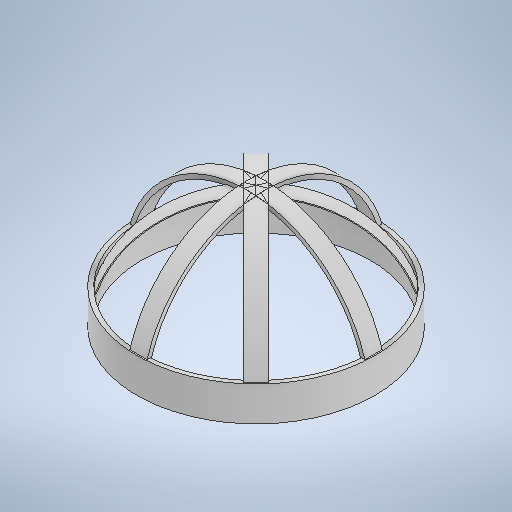
# Autodesk Inventor part: Original Dome
Saved by Autodesk Inventor 2025.1 (Build 291241000, 241)
## iProperties
Created: 2024-11-11
Part Number: Original Dome
Material: Generic
Document SubType Name: Modeling
Designer: monos
Density: 1 g/cm^3
Appearance: Default
Author: monos
Autodesk Inventor part; units mm, degrees
ref_plane "XZ Plane" through (0, 0, 0) normal (0, 1, 0) x (-1, 0, 0)
sketch "Sketch1" plane through (0, 0, 0) normal (0, 1, 0) x (-1, 0, 0)
  circle A0 centre (0, 0) radius 87.5
  circle A1 centre (0, 0) radius 84.325
  dimension "d0" = 175
  dimension "d1" = 168.65
  constraints: 2 centre point, 2 coincident
  measures "d0" diameter of A0
  measures "d1" diameter of A1
extrude "Extrusion1" add sketch "Sketch1" along normal blind 25.4
sketch "Sketch2" plane through (0, 0, 0) normal (1, 0, 0) x (0, 1, 0)
  point P0 (0, 0)
ref_plane "Work Plane1" through (0, 0, 0) normal (0.7071068, 0, -0.7071068) x (0, 1, 0)
sketch "Sketch5" plane through (0, 0, 0) normal (0.7071068, 0, -0.7071068) x (0, 1, 0)
  line L0 (0, -87.5) -> (0, 87.5) projected
  arc A0 (25.4, -86.3414) -> (90, 0) centre (0, 0) ccw
  arc A1 (90, 0) -> (25.4, 86.3414) centre (0, 0) ccw
  arc A2 (25.4, -83.0266) -> (86.825, 0) centre (0, 0) ccw
  arc A3 (86.825, 0) -> (25.4, 83.0266) centre (0, 0) ccw
  line L1 (90, 0) -> (86.825, 0)
  line L2 (25.4187, -86.3359) -> (25.4, -83.0266)
  line L3 (25.4, -87.5) -> (25.4, 87.5) projected
  line L4 (25.4, 83.0266) -> (25.4, 86.3414)
  point P0 (86.825, 0)
  dimension "d13" = 86.825
  dimension "d14" = 86.825
  constraints: 9 point on circle, 6 end point, 4 centre point, 4 coincident, 4 point on line, 1 horizontal
  measures "d13" radius of A2
  measures "d14" radius of A3
extrude "Extrusion4" add sketch "Sketch5" along normal mid plane 12.7 contours L2 A2 L1 A0 | L1 A3 L3 A1
sketch "Sketch3" plane through (0, 0, 0) normal (1, 0, 0) x (0, 1, 0)
  line L0 (0, -87.5) -> (0, 87.5) projected
  arc A0 (90, 0) -> (25.4046, 86.3401) centre (0, 0) ccw
  arc A1 (25.428, -86.3332) -> (90, 0) centre (0, 0) ccw
  arc A2 (25.428, -83.018) -> (86.825, 0) centre (0, 0) ccw
  line L1 (86.825, 0) -> (90, 0)
  line L2 (25.428, -83.018) -> (25.428, -86.3332)
  arc A3 (86.825, 0) -> (25.4046, 83.0252) centre (0, 0) ccw
  line L3 (90, 0) -> (86.825, 0)
  line L4 (25.4046, 86.3401) -> (25.4046, 83.0252)
  dimension "d5" = 86.825
  dimension "d6" = 86.825
  constraints: 8 end point, 8 point on circle, 4 centre point, 4 coincident, 2 horizontal, 1 perpendicular, 1 vertical
  measures "d5" radius of A2
  measures "d6" radius of A3
extrude "Extrusion2" add sketch "Sketch3" along normal mid plane 12.7
sketch "Sketch4" plane through (0, 0, 0) normal (0, 0, 1) x (1, 0, 0)
  line L0 (87.5, 0) -> (-87.5, 0) projected
  arc A0 (0, 90) -> (-86.3414, 25.4) centre (0, 0) ccw
  arc A1 (0, 86.825) -> (-83.0266, 25.4) centre (0, 0) ccw
  arc A2 (83.0266, 25.4) -> (0, 86.825) centre (0, 0) ccw
  line L1 (83.0266, 25.4) -> (86.3414, 25.4)
  line L2 (-86.3414, 25.4) -> (-83.0266, 25.4)
  arc A3 (86.3414, 25.4) -> (0, 90) centre (0, 0) ccw
  line L3 (0, 90) -> (0, 86.825)
  line L4 (0, 90) -> (0, 86.825)
  line L5 (83.0266, 25.4) -> (86.3414, 25.4)
  ellipse E0 centre (4.4901, 0) end of major axis (4.4901, 90) minor radius 63.6396 (-6.35, 88.6847) -> (-56.5586, 25.4187) ccw projected
  line L6 (-83.0266, 25.4) -> (-86.3414, 25.4)
  dimension "d9" = 86.825
  dimension "d10" = 86.825
  constraints: 12 end point, 8 point on circle, 4 centre point, 4 coincident, 2 vertical, 1 collinear, 1 horizontal, 1 other
  measures "d9" radius of A1
  measures "d10" radius of A2
extrude "Extrusion5" add sketch "Sketch4" along normal mid plane 12.7
ref_plane "Work Plane3" through (0, 0, 0) normal (0.7071068, 0, 0.7071068) x (0, 1, 0)
sketch "Sketch6" plane through (0, 0, 0) normal (0.7071068, 0, 0.7071068) x (0, 1, 0)
  line L0 (0, -87.5) -> (0, 87.5) projected
  arc A0 (87.5, 0) -> (0, 87.5) centre (0, 0) ccw
  arc A1 (0, -87.5) -> (87.5, 0) centre (0, 0) ccw
  arc A2 (86.825, 0) -> (0, 86.825) centre (0, 0) ccw
  arc A3 (0, -86.825) -> (86.825, 0) centre (0, 0) ccw
  line L1 (87.5, 0) -> (86.825, 0)
  line L2 (24.6994, 83.9416) -> (25.4, 83.0266)
  line L3 (25.4, 84.325) -> (25.4, -84.325) projected
  line L4 (25.4, -83.0266) -> (25.4, -83.7323)
  dimension "d19" = 86.825
  dimension "d20" = 86.825
  constraints: 12 point on circle, 6 end point, 4 centre point, 4 coincident, 4 point on line, 1 horizontal
  measures "d19" radius of A2
  measures "d20" radius of A3
extrude "Extrusion6" add sketch "Sketch6" along normal mid plane 12.7 contours L3 A3 L1 A1 | L1 A2 L3 A0 | L2 A0 L3
body "Solid1"
